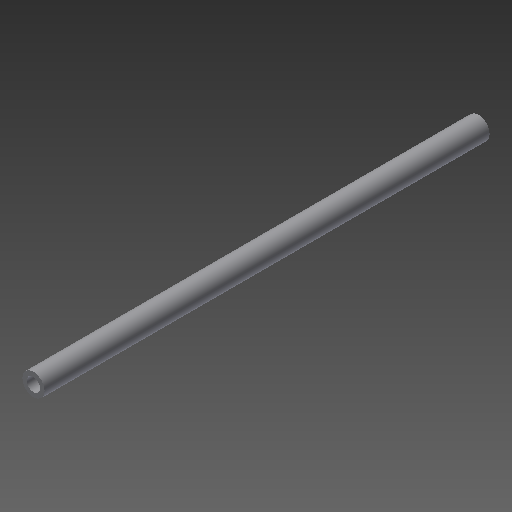
# Autodesk Inventor part: 3d_LM - Tubo 1x1
Saved by Autodesk Inventor 2018.3 (Build 223284000, 284)
## iProperties
Created: 2025-09-03
Part Number: 3d_LM - Tubo 1x1
Material: Genérico
Document SubType Name: Modeling
Designer: mbs18
Density: 1 g/cm^3
Appearance: Valor por defecto
Manufacturer-1: {"Name": "\nEmbention Sistemas Inteligentes S.A.", "PartNumber": "3d_LM - Tubo 1x1", "Link": ""}
Manufacturer-2: {"Name": "", "PartNumber": "", "Link": ""}
Manufacturer-3: {"Name": "", "PartNumber": "", "Link": ""}
Manufacturer-4: {"Name": "", "PartNumber": "", "Link": ""}
Manufacturer-5: {"Name": "", "PartNumber": "", "Link": ""}
Provider-1: {"Name": "", "PartNumber": "", "Link": ""}
Provider-2: {"Name": "", "PartNumber": "", "Link": ""}
Provider-3: {"Name": "", "PartNumber": "", "Link": ""}
Provider-4: {"Name": "", "PartNumber": "", "Link": ""}
Provider-5: {"Name": "", "PartNumber": "", "Link": ""}
Author: mbs18
Autodesk Inventor part; units mm, degrees
ref_plane "YZ Plane" through (0, 0, 0) normal (1, 0, 0) x (0, 1, 0)
ref_plane "XZ Plane" through (0, 0, 0) normal (0, 1, 0) x (-1, 0, 0)
ref_plane "XY Plane" through (0, 0, 0) normal (0, 0, 1) x (1, 0, 0)
sketch "Sketch1" plane through (0, 0, 0) normal (0, 0, 1) x (1, 0, 0)
  circle A0 centre (0, 0) radius 1
  circle A1 centre (0, 0) radius 0.6
  dimension "d0" = 2
  dimension "d1" = 1.2
  constraints: 2 centre point, 2 coincident
  measures "d0" diameter of A0
  measures "d1" diameter of A1
extrude "Extrusion1" add sketch "Sketch1" along normal blind 40
body "Solid1"
